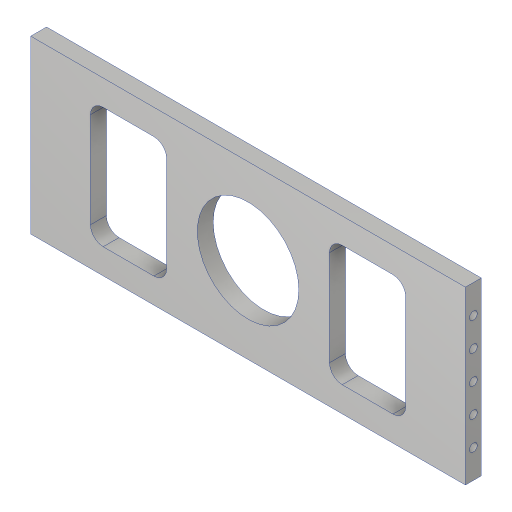
# Autodesk Inventor part: J2L1_H_Top
Saved by Autodesk Inventor 2023.2 (Build 272271000, 271)
## iProperties
Created: 2021-07-07
Part Number: J2L1_H_Top
Material: 알루미늄 6061
Document SubType Name: Modeling
Designer: user
Density: 2.7 g/cm^3
Appearance: 알루미늄 - 평지
Mass: 82.68 g
Surface Area: 166.428 cm^2
Volume: 30.6222 cm^3
Author: user
Autodesk Inventor part; units mm, degrees
ref_plane "YZ Plane" through (0, 0, 0) normal (1, 0, 0) x (0, 1, 0)
ref_plane "XZ Plane" through (0, 0, 0) normal (0, 1, 0) x (-1, 0, 0)
ref_plane "XY Plane" through (0, 0, 0) normal (0, 0, 1) x (1, 0, 0)
sketch "스케치1" plane through (0, 0, 0) normal (0, 0, 1) x (1, 0, 0)
  line L0 (-68.5, 27) -> (68.5, 27)
  line L1 (68.5, 27) -> (68.5, -27)
  line L2 (68.5, -27) -> (-68.5, -27)
  line L3 (-68.5, -27) -> (-68.5, 27)
  point P0 (0, 0)
  dimension "d0" = 137
  dimension "d1" = 54
  dimension "d2" = 27
  dimension "d3" = 68.5
  constraints: 8 end point, 2 parallel, 1 horizontal, 1 perpendicular
  measures "d0" distance of L1.end L2.end
  measures "d1" distance of L0.end L1.end
  measures "d2" distance from line of L0 point (0, 0)
  measures "d3" distance from line of L3 point (0, 0)
extrude "돌출1" add sketch "스케치1" along normal blind 5
sketch "스케치2" plane through (-68.5, -27, 0) normal (-1, 0, 0) x (0, 0, 1)
  line L0 (0, 54) -> (0, 0)
  line L1 (0, 0) -> (5, 0)
  line L2 (5, 0) -> (51, 4)
  line L3 (51, 50) -> (5, 54)
  line L4 (5, 54) -> (0, 54)
  circle A0 centre (2.5, 9) radius 1.25
  circle A1 centre (2.5, 18) radius 1.25
  circle A2 centre (2.5, 27) radius 1.25
  circle A3 centre (2.5, 36) radius 1.25
  circle A4 centre (2.5, 45) radius 1.25
  line L5 (0, 0) -> (0, 54) projected
  line L6 (0, 0) -> (5, 0) projected
  line L7 (5, 54) -> (5, 0) projected
  line L8 (0, 54) -> (5, 54) projected
  point P0 (0, 27)
  dimension "d6" = 2.5
  dimension "d7" = 2.5
  dimension "d8" = 2.5
  dimension "d9" = 2.5
  dimension "d10" = 2.5
  dimension "d11" = 2.5
  dimension "d12" = 2.5
  dimension "d13" = 2.5
  dimension "d14" = 2.5
  dimension "d15" = 2.5
  dimension "d16" = 9
  dimension "d17" = 18
  dimension "d18" = 27
  dimension "d19" = 36
  dimension "d20" = 9
  constraints: 10 end point, 5 centre point
  measures "d6" diameter of A0
  measures "d7" distance from line of L0 A0.centre
  measures "d8" diameter of A1
  measures "d9" diameter of A2
  measures "d10" diameter of A3
  measures "d11" diameter of A4
  measures "d12" distance from line of L0 A1.centre
  measures "d13" distance from line of L0 A2.centre
  measures "d14" distance from line of L0 A3.centre
  measures "d15" distance from line of L0 A4.centre
  measures "d16" distance from line of L1 A0.centre
  measures "d17" distance from line of L1 A1.centre
  measures "d18" distance from line of L1 A2.centre
  measures "d19" distance from line of L1 A3.centre
  measures "d20" distance from line of L4 A4.centre
extrude "돌출2" cut sketch "스케치2" against normal blind 10 contours A0 | A1 | A2 | A3 | A4
sketch "스케치3" plane through (68.5, -27, 0) normal (1, 0, 0) x (0, 0, -1)
  line L0 (0, 0) -> (0, 54)
  line L1 (0, 54) -> (-5, 54)
  line L2 (-5, 54) -> (-51, 50)
  line L3 (-51, 4) -> (-5, 0)
  line L4 (-5, 0) -> (0, 0)
  circle A0 centre (-2.5, 45) radius 1.25
  circle A1 centre (-2.5, 36) radius 1.25
  circle A2 centre (-2.5, 27) radius 1.25
  circle A3 centre (-2.5, 18) radius 1.25
  circle A4 centre (-2.5, 9) radius 1.25
  line L5 (0, 54) -> (0, 0) projected
  line L6 (0, 54) -> (-5, 54) projected
  line L7 (-5, 0) -> (-5, 54) projected
  line L8 (0, 0) -> (-5, 0) projected
  point P0 (0, 27)
  dimension "d23" = 2.5
  dimension "d24" = 2.5
  dimension "d25" = 2.5
  dimension "d26" = 2.5
  dimension "d27" = 2.5
  dimension "d28" = 2.5
  dimension "d29" = 2.5
  dimension "d30" = 2.5
  dimension "d31" = 2.5
  dimension "d32" = 2.5
  dimension "d33" = 9
  dimension "d34" = 18
  dimension "d35" = 27
  dimension "d36" = 36
  dimension "d37" = 9
  constraints: 10 end point, 5 centre point
  measures "d23" diameter of A0
  measures "d24" distance from line of L0 A0.centre
  measures "d25" diameter of A1
  measures "d26" diameter of A2
  measures "d27" diameter of A3
  measures "d28" diameter of A4
  measures "d29" distance from line of L0 A1.centre
  measures "d30" distance from line of L0 A2.centre
  measures "d31" distance from line of L0 A3.centre
  measures "d32" distance from line of L0 A4.centre
  measures "d33" distance from line of L1 A0.centre
  measures "d34" distance from line of L1 A1.centre
  measures "d35" distance from line of L1 A2.centre
  measures "d36" distance from line of L1 A3.centre
  measures "d37" distance from line of L4 A4.centre
extrude "돌출3" cut sketch "스케치3" against normal blind 10 contours A0 | A1 | A2 | A3 | A4
sketch "스케치5" plane through (0, 0, 5) normal (0, 0, 1) x (1, 0, 0)
  line L0 (68.5, 27) -> (-68.5, 27) projected
  line L1 (-68.5, 27) -> (-68.5, -27) projected
  line L2 (-68.5, -27) -> (68.5, -27) projected
  line L3 (68.5, -27) -> (68.5, 27) projected
  line L4 (68.5, 27) -> (-68.5, 27) projected
  line L5 (-68.5, -0.0341) -> (68.5, 0) construction
  line L6 (-45.6619, 19) -> (-29.6619, 19)
  line L7 (-25.6619, 15) -> (-25.6619, -15.0528)
  line L8 (-29.6619, -19.0528) -> (-45.6619, -19.0528)
  line L9 (-49.6619, -15.0528) -> (-49.6619, 15)
  line L10 (-49.6619, 19) -> (-25.6619, -19.0528) construction
  line L11 (-25.6619, 19) -> (-49.6619, -19.0528) construction
  arc A0 (-45.6619, 19) -> (-49.6619, 15) centre (-45.6619, 15) ccw
  arc A1 (-25.6619, 15) -> (-29.6619, 19) centre (-29.6619, 15) ccw
  arc A2 (-29.6619, -19.0528) -> (-25.6619, -15.0528) centre (-29.6619, -15.0528) ccw
  arc A3 (-49.6619, -15.0528) -> (-45.6619, -19.0528) centre (-45.6619, -15.0528) ccw
  line L12 (0, 29) -> (0, -29)
  arc A4 (29.6619, 19) -> (25.6619, 15) centre (29.6619, 15) ccw
  line L13 (25.6619, 15) -> (25.6619, -15.0528)
  arc A5 (25.6619, -15.0528) -> (29.6619, -19.0528) centre (29.6619, -15.0528) ccw
  line L14 (45.6619, 19) -> (29.6619, 19)
  arc A6 (49.6619, 15) -> (45.6619, 19) centre (45.6619, 15) ccw
  line L15 (49.6619, 19) -> (25.6619, -19.0528) construction
  line L16 (25.6619, 19) -> (49.6619, -19.0528) construction
  line L17 (49.6619, -15.0528) -> (49.6619, 15)
  arc A7 (45.6619, -19.0528) -> (49.6619, -15.0528) centre (45.6619, -15.0528) ccw
  line L18 (29.6619, -19.0528) -> (45.6619, -19.0528)
  point P0 (0, 0)
  point P1 (-37.6619, -0.0264)
  point P2 (37.6619, -0.0264)
  point P3 (0, 0)
  dimension "d85" = 24
  dimension "d86" = 4
  constraints: 28 end point, 17 point on line, 16 point on circle, 8 centre point, 8 tangent, 3 equal radius, 3 midpoint, 2 parallel, 1 horizontal, 1 perpendicular
  measures "d85" distance of L10.end L11.end
  measures "d86" radius of A0
extrude "돌출4" cut sketch "스케치5" against normal up to surface (5 mm away) contours L6 A1 L7 A2 L8 A3 L9 A0 | L14 A6 L17 A7 L18 A5 L13 A4
sketch "스케치9" plane through (0, 0, 5) normal (0, 0, 1) x (1, 0, 0)
  circle A0 centre (0, 0) radius 16
  dimension "d82" = 32
  constraints: 1 centre point, 1 coincident
  measures "d82" diameter of A0
extrude "돌출8" cut sketch "스케치9" against normal blind 10
equation "\"d2\" = 0.5 * d1"
equation "\"d3\" = 0.5 * d0"
